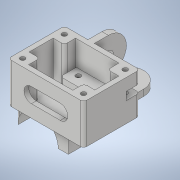
# Autodesk Inventor part: Caixa dianteira
Saved by Autodesk Inventor 2021 (Build 250183000, 183)
## iProperties
Created: 2021-05-27
Part Number: Caixa dianteira
Material: Generic
Document SubType Name: Modeling
Designer: hoope
Density: 1 g/cm^3
Appearance: Default
Author: hoope
Autodesk Inventor part; units mm, degrees
ref_plane "YZ Plane" through (0, 0, 0) normal (1, 0, 0) x (0, 1, 0)
ref_plane "XZ Plane" through (0, 0, 0) normal (0, 1, 0) x (-1, 0, 0)
ref_plane "XY Plane" through (0, 0, 0) normal (0, 0, 1) x (1, 0, 0)
sketch "Esboço1" plane through (0, 0, 0) normal (0, 1, 0) x (-1, 0, 0)
  line L0 (0, 0) -> (47, 0)
  line L1 (47, 0) -> (47, 35)
  line L2 (47, 35) -> (0, 35)
  line L3 (0, 35) -> (0, 0)
  dimension "d0" = 47
  dimension "d1" = 35
  constraints: 8 end point, 2 parallel, 1 horizontal, 1 perpendicular
  measures "d0" distance of L2.end L1.end
  measures "d1" distance of L1.end L0.end
extrude "Extrusão1" add sketch "Esboço1" along normal blind 25
shell "Casca1" thickness 3 removed faces 1 at (-15.6667, 25, 23.3333)
sketch "Esboço2" plane through (-47, 0, 35) normal (0, 0, 1) x (1, 0, 0)
  arc A0 (14.5, 17.15) -> (14.5, 7.85) centre (14.5, 12.5) ccw
  line L0 (0, 25) -> (47, 25) projected
  arc A1 (32.5, 7.85) -> (32.5, 17.15) centre (32.5, 12.5) ccw
  line L1 (47, 0) -> (47, 25) projected
  line L2 (14.5, 17.15) -> (32.5, 17.15)
  line L3 (32.5, 7.85) -> (14.5, 7.85)
  dimension "d5" = 9.3
  dimension "d6" = 12.5
  dimension "d7" = 9.3
  dimension "d8" = 18
  dimension "d9" = 14.5
  constraints: 4 end point, 4 point on circle, 2 centre point, 1 horizontal, 1 parallel
  measures "d5" diameter of A0
  measures "d6" distance from line of L0 A0.centre
  measures "d7" diameter of A1
  measures "d8" distance of A1.centre A0.centre
  measures "d9" distance from line of L1 A1.centre
extrude "Extrusão2" cut sketch "Esboço2" against normal blind 10
sketch "Esboço3" plane through (-44, 3, 3) normal (0, 1, 0) x (1, 0, 0)
  line L0 (41, 0) -> (0, 0) projected
  line L1 (0, 0) -> (7, 0)
  line L2 (7, 0) -> (7, -7)
  line L3 (7, -7) -> (0, -7)
  line L4 (0, -7) -> (0, 0)
  line L5 (41, 0) -> (34, 0)
  line L6 (34, 0) -> (34, -7)
  line L7 (34, -7) -> (41, -7)
  line L8 (41, -7) -> (41, 0)
  line L9 (41, -29) -> (34.3, -29)
  line L10 (34.3, -29) -> (34.3, -22)
  line L11 (34.3, -22) -> (41, -22)
  line L12 (41, -22) -> (41, -29)
  line L13 (41, -29) -> (0, -29) projected
  line L14 (0, -29) -> (6.7, -29)
  line L15 (6.7, -29) -> (6.7, -22)
  line L16 (6.7, -22) -> (0, -22)
  line L17 (0, -22) -> (0, -29)
  point P0 (44, 3)
  dimension "d12" = 7
  dimension "d13" = 7
  dimension "d14" = 7
  dimension "d15" = 7
  dimension "d16" = 6.7
  dimension "d17" = 7
  dimension "d18" = 6.7
  dimension "d19" = 7
  constraints: 32 end point, 8 parallel, 4 horizontal, 4 perpendicular
  measures "d12" distance of L2.end L3.end
  measures "d13" distance of L1.end L2.end
  measures "d14" distance of L7.end L6.end
  measures "d15" distance of L6.end L5.end
  measures "d16" distance of L10.end L11.end
  measures "d17" distance of L9.end L10.end
  measures "d18" distance of L16.end L15.end
  measures "d19" distance of L15.end L14.end
extrude "Extrusão3" add sketch "Esboço3" along normal blind 22
sketch "Esboço4" plane through (-37, 3, 3) normal (0, 1, 0) x (1, 0, 0)
  line L0 (27, 0) -> (27, -7) projected
  line L1 (0, -7) -> (0, 0) projected
  line L2 (0, 0) -> (27, 0) projected
  line L3 (27, 0) -> (0, 0) projected
  line L4 (0.5, 0) -> (26.5, 0)
  line L5 (26.5, 0) -> (26.5, -10)
  line L6 (26.5, -10) -> (0.5, -10)
  line L7 (0.5, -10) -> (0.5, 0)
  line L8 (5.72, -0.65) -> (8.6212, -2.325)
  line L9 (8.6212, -2.325) -> (8.6212, -5.675)
  line L10 (8.6212, -5.675) -> (5.72, -7.35)
  line L11 (5.72, -7.35) -> (2.8188, -5.675)
  line L12 (2.8188, -5.675) -> (2.8188, -2.325)
  line L13 (2.8188, -2.325) -> (5.72, -0.65)
  line L14 (21.28, -0.65) -> (24.1812, -2.325)
  line L15 (24.1812, -2.325) -> (24.1812, -5.675)
  line L16 (24.1812, -5.675) -> (21.28, -7.35)
  line L17 (21.28, -7.35) -> (18.3788, -5.675)
  line L18 (18.3788, -5.675) -> (18.3788, -2.325)
  line L19 (18.3788, -2.325) -> (21.28, -0.65)
  point P0 (37, 3)
  point P1 (5.72, -4)
  point P2 (21.28, -4)
  dimension "d33" = 26
  dimension "d34" = 10
  constraints: 32 end point, 2 parallel, 1 horizontal, 1 perpendicular, 1 point on line, 26 other
  measures "d33" distance between parallel lines of L5 L7
  measures "d34" distance between parallel lines of L4 L6
fillet "Arredondamento1" radius 2 4 edges at (-47, 12.5, 35) (0, 12.5, 35) (0, 12.5, 0) (-47, 12.5, 0)
fillet "Arredondamento2" radius 2 4 edges at (-37, 14, 10) (-10, 14, 10) (-37.3, 14, 25) (-9.7, 14, 25)
sketch "Esboço14" plane through (-2, 0, 0) normal (0, 0, -1) x (-1, 0, 0)
  arc A0 (44.2, -13) -> (18.8, -13) centre (31.5, -13) ccw
  line L0 (0, 0) -> (43, 0) projected
  line L1 (45, 0) -> (45, 25) projected
  line L2 (45, 0) -> (45, -13)
  line L3 (45, -13) -> (44.2, -13)
  line L4 (18.8, -13) -> (17.5, -13)
  line L5 (45, 0) -> (43, 0) projected
  line L6 (12.5, 0) -> (45, 0)
  line L7 (17.5, -13) -> (12.5, -13)
  line L8 (12.5, -13) -> (12.5, 0)
  line L9 (12.5, 0) -> (12.5, 0)
  point P0 (-2, 0)
  dimension "d97" = 25.4
  dimension "d98" = 13
  dimension "d99" = 13.5
  dimension "d100" = 1.3
  dimension "d176" = 5
  constraints: 14 end point, 2 collinear, 2 horizontal, 2 perpendicular, 2 point on circle, 2 point on line, 1 centre point, 1 vertical
  measures "d97" diameter of A0
  measures "d98" distance from line of L0 A0.centre
  measures "d99" distance from line of L1 A0.centre
  measures "d100" distance of L4.start L4.end
  measures "d176" distance of L4.end L7.end
extrude "Extrusão12" add sketch "Esboço14" against normal blind 30
fillet "Arredondamento5" radius 2 2 edges at (-47, -6.5, 0) (-47, -6.5, 30)
sketch "Esboço15" plane through (-2, 25, 0) normal (0, 0, -1) x (-1, 0, 0)
  line L0 (26.3, 0) -> (30.3, 0)
  line L1 (30.3, 0) -> (30.3, -22)
  line L2 (30.3, -22) -> (26.3, -22)
  line L3 (26.3, -22) -> (26.3, 0)
  line L4 (0, 0) -> (43, 0) projected
  line L5 (45, -38) -> (45, 0) projected
  point P0 (-2, -25)
  dimension "d104" = 4
  dimension "d105" = 22
  dimension "d106" = 0
  dimension "d107" = 14.7
  constraints: 8 end point, 2 parallel, 1 horizontal, 1 perpendicular
  measures "d104" distance of L1.end L2.end
  measures "d105" distance of L0.end L1.end
  measures "d106" distance between parallel lines of L4 L0
  measures "d107" distance between parallel lines of L5 L1
extrude "Extrusão13" add sketch "Esboço15" along normal blind 20
fillet "Arredondamento6" radius 11.25 2 edges at (-30.3, 25, -20) (-30.3, 3, -20)
sketch "Esboço27" plane through (-2, 25, 0) normal (0, 0, -1) x (-1, 0, 0)
  line L0 (5.487, -23.2) -> (25.487, -23.2)
  line L1 (25.487, -23.2) -> (25.487, -19.2)
  line L2 (25.487, -19.2) -> (5.487, -19.2)
  line L3 (5.487, -19.2) -> (5.487, -23.2)
  line L4 (0, -25) -> (12.5, -25) projected
  line L5 (-2, 0) -> (-2, -25) projected
  point P0 (12.5, -25)
  dimension "d143" = 20
  dimension "d144" = 4
  dimension "d156" = 1.8
  dimension "d157" = 7.487
  constraints: 8 end point, 2 parallel, 1 horizontal, 1 perpendicular
  measures "d143" distance of L2.end L1.end
  measures "d144" distance of L1.end L0.end
  measures "d156" distance between parallel lines of L4 L0
  measures "d157" distance between parallel lines of L5 L3
extrude "Extrusão23" add sketch "Esboço27" along normal blind 20
fillet "Arredondamento8" radius 10 2 edges at (-7.487, 3.8, -20) (-27.487, 3.8, -20)
sketch "Esboço29" plane through (-27.487, 5.8, 0) normal (0, 1, 0) x (1, 0, 0)
  arc A0 (20, 10) -> (0, 10) centre (10, 10) ccw projected
  circle A1 centre (10, 10) radius 3
  point P0 (27.487, 0)
  dimension "d150" = 6
  constraints: 1 centre point, 1 coincident
  measures "d150" diameter of A1
extrude "Extrusão24" cut sketch "Esboço29" against normal blind 20
sketch "Esboço30" plane through (-28.3, 3, 0) normal (1, 0, 0) x (0, 0, -1)
  arc A0 (20, 10.75) -> (8.75, 22) centre (8.75, 10.75) ccw projected
  circle A1 centre (8.75, 10.75) radius 3
  point P0 (0, -3)
  dimension "d153" = 6
  constraints: 1 centre point, 1 coincident
  measures "d153" diameter of A1
extrude "Extrusão25" cut sketch "Esboço30" against normal blind 20
sketch "Esboço36" plane through (0, 25, 0) normal (0, 1, 0) x (1, 0, 0)
  circle A0 centre (-4.5, -4.5) radius 1.505
  line L0 (-2, 0) -> (-28.3, 0) projected
  line L1 (0, -33) -> (0, -2) projected
  circle A1 centre (-4.5, -30.5) radius 1.505
  circle A2 centre (-42.5, -4.5) radius 1.505
  circle A3 centre (-42.5, -30.5) radius 1.505
  point P0 (0, 0)
  dimension "d184" = 3.01
  dimension "d185" = 4.5
  dimension "d186" = 4.5
  dimension "d189" = 26
  dimension "d192" = 38
  constraints: 4 centre point, 1 horizontal, 1 vertical, 6 other
  measures "d184" diameter of A0
  measures "d185" distance from line of L0 A0.centre
  measures "d186" distance from line of L1 A0.centre
  measures "d189" distance of A0.centre A1.centre
  measures "d192" distance of A0.centre A2.centre
extrude "Extrusão28" cut sketch "Esboço36" against normal blind 19
sketch "Esboço37" plane through (0, 0, 33) normal (1, 0, 0) x (0, 0, -1)
  line L0 (33, 25) -> (33, -7.6111) projected
  line L1 (33, 17.5) -> (24.5, 17.5)
  line L2 (24.5, 17.5) -> (24.5, 12.5)
  line L3 (24.5, 12.5) -> (33, 12.5)
  line L4 (33, 12.5) -> (33, 17.5)
  line L5 (0, 25) -> (31, 25) projected
  point P0 (33, 0)
  dimension "d197" = 8.5
  dimension "d198" = 5
  dimension "d199" = 7.5
  constraints: 8 end point, 2 parallel, 1 horizontal, 1 perpendicular, 1 point on line
  measures "d197" distance of L3.end L2.end
  measures "d198" distance of L2.end L1.end
  measures "d199" distance between parallel lines of L5 L1
extrude "Extrusão29" cut sketch "Esboço37" against normal blind 8.5
sketch "Esboço38" plane through (-47, 0, 33) normal (-1, 0, 0) x (0, 0, 1)
  line L0 (-33, 0) -> (-33, 12.5) projected
  line L1 (-33, 12.5) -> (-24.5, 12.5)
  line L2 (-24.5, 12.5) -> (-24.5, 17.5)
  line L3 (-24.5, 17.5) -> (-33, 17.5)
  line L4 (-33, 17.5) -> (-33, 12.5)
  line L5 (-31, 25) -> (0, 25) projected
  dimension "d202" = 8.5
  dimension "d203" = 5
  dimension "d204" = 7.5
  constraints: 8 end point, 2 parallel, 1 horizontal, 1 perpendicular, 1 point on line
  measures "d202" distance of L3.end L2.end
  measures "d203" distance of L2.end L1.end
  measures "d204" distance between parallel lines of L5 L3
extrude "Extrusão30" cut sketch "Esboço38" against normal blind 8.5
extrude "Extrusão31" add sketch "Esboço4" along normal blind 4.5
sketch "Esboço40" plane through (-37, 7.5, 3) normal (0, 1, 0) x (1, 0, 0)
  line L0 (0.5, 0) -> (0, 0) projected
  line L1 (26.5, -10) -> (0.5, -10) projected
  line L2 (0.5, 0) -> (26.5, 0)
  line L3 (26.5, 0) -> (26.5, -10)
  line L4 (26.5, -10) -> (0.5, -10)
  line L5 (0.5, -10) -> (0.5, 0)
  point P0 (37, 3)
  constraints: 8 end point, 2 parallel, 1 horizontal, 1 perpendicular
extrude "Extrusão32" add sketch "Esboço40" along normal blind 2
sketch "Esboço41" plane through (-37, 9.5, 3) normal (0, 1, 0) x (1, 0, 0)
  circle A0 centre (5.72, -4) radius 1.55
  circle A1 centre (21.28, -4) radius 1.505
  point P0 (37, 3)
  dimension "d215" = 3.1
  dimension "d216" = 3.01
  constraints: 2 centre point
  measures "d215" diameter of A0
  measures "d216" diameter of A1
extrude "Extrusão33" cut sketch "Esboço41" against normal blind 2
chamfer "Chanfro5" distance 1.5 angle 45 2 edges at (-10.5, 6.25, 13) (-36.5, 6.25, 13)
